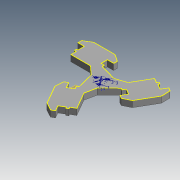
# Autodesk Inventor part: Part2
Saved by Autodesk Inventor 2014 SP1 (Build 180222100, 222)
## iProperties
Created: 2014-04-03
Part Number: Part2
Material: Generic
Document SubType Name: Modeling
Designer: tom
Density: 1 g/cm^3
Appearance: Default
Author: tom
Autodesk Inventor part; units mm, degrees
ref_plane "YZ Plane" through (0, 0, 0) normal (1, 0, 0) x (0, 1, 0)
ref_plane "XZ Plane" through (0, 0, 0) normal (0, 1, 0) x (-1, 0, 0)
ref_plane "XY Plane" through (0, 0, 0) normal (0, 0, 1) x (1, 0, 0)
ref_plane "Work Plane3" through (-98.2192, 25.6748, -72.651) normal (0, 1, 0) x (1, 0, 0)
sketch "Sketch1" plane through (-98.2192, 25.6748, -72.651) normal (0, 1, 0) x (1, 0, 0)
  line L0 (108.2722, -112.7231) -> (109.1382, -112.2231) construction
  line L1 (108.6382, -111.3571) -> (109.1382, -112.2231) construction
  line L2 (101.5917, -99.1522) -> (114.8917, -122.1885)
  line L3 (114.8917, -122.1885) -> (108.6563, -125.7885)
  line L4 (108.6563, -125.7885) -> (109.9613, -128.0488)
  line L5 (109.9613, -128.0488) -> (107.3632, -129.5488)
  line L6 (107.3632, -129.5488) -> (106.3632, -127.8168)
  line L7 (106.3632, -127.8168) -> (98.8635, -132.1468)
  line L8 (98.8635, -132.1468) -> (103.1935, -139.6466)
  line L9 (79.4712, -121.2385) -> (82.4842, -126.4571) construction
  line L10 (103.1935, -139.6466) -> (98.8633, -142.1466)
  line L11 (83.0235, -104.7111) -> (90.5232, -100.3811)
  line L12 (90.5232, -100.3811) -> (88.3182, -96.5619)
  line L13 (88.3182, -96.5619) -> (90.8427, -95.1044)
  line L14 (83.0235, -104.7111) -> (78.6935, -97.2113)
  line L15 (73.6327, -111.1259) -> (88.2377, -136.4225)
  line L16 (78.6935, -97.2113) -> (74.3633, -99.7113)
  line L17 (90.8427, -95.1044) -> (85.0892, -72.651)
  line L18 (104.7842, -84.0219) -> (98.2192, -72.651)
  line L19 (98.2192, -72.651) -> (85.0892, -72.651)
  line L20 (88.2377, -136.4225) -> (98.8633, -142.1466)
  line L21 (74.3633, -99.7113) -> (73.6327, -111.1259)
  line L22 (98.2192, -72.651) -> (104.7842, -84.0219)
  line L23 (104.7842, -84.0219) -> (101.5917, -99.1522)
  dimension "d1" = 26.6
  dimension "d4" = 7.2
  dimension "d5" = 2.61
  dimension "d6" = 3
  dimension "d7" = 2
  dimension "d8" = 8.66
  dimension "d9" = 8.66
  dimension "d10" = 5
  dimension "d11" = 8.66
  dimension "d12" = 31.68
  dimension "d13" = 4.41
  dimension "d14" = 2.915
  dimension "d17" = 8.66
  dimension "d18" = 29.21
  dimension "d20" = 10.27
  dimension "d21" = 5
  dimension "d22" = 23.1789
  dimension "d23" = 13.13
  dimension "d31" = 13.13
  constraints: 48 end point, 7 perpendicular, 1 collinear, 1 parallel
  measures "d1" distance of L2.start L2.end
  measures "d4" distance of L2.end L3.end
  measures "d5" distance of L3.end L4.end
  measures "d6" distance of L4.end L5.end
  measures "d7" distance of L5.end L6.end
  measures "d8" distance of L6.end L7.end
  measures "d9" distance of L7.end L8.end
  measures "d10" distance of L8.end L10.end
  measures "d11" distance of L11.start L11.end
  measures "d12" distance between parallel lines of L7 L11
  measures "d13" distance of L11.end L12.end
  measures "d14" distance of L12.end L13.end
  measures "d17" distance of L11.start L14.end
  measures "d18" distance of L15.start L15.end
  measures "d20" distance from line of L10 L15.end
  measures "d21" distance of L14.end L16.end
  measures "d22" distance of L13.end L17.end
  measures "d23" distance of L18.end L17.end
  measures "d31" distance of L18.start L18.end
extrude "Extrusion1" add sketch "Sketch1" along normal blind 8.66
pattern_circular "Circular Pattern2" count 3 over 360 about axis through (0, 25.6748, 0) along (0, 1, 0) of "Extrusion1"
sketch "Sketch2" plane through (-98.2192, 34.3348, -72.651) normal (0, 1, 0) x (1, 0, 0)
  line L0 (46.9822, -62.321) -> (73.5822, -62.321) projected
  line L1 (114.8917, -122.1885) -> (101.5917, -99.1522) projected
  circle A0 centre (98.2192, -72.651) radius 1.5
  line L2 (98.2192, -72.651) -> (104.7842, -84.0219) construction
  line L3 (98.2192, -72.651) -> (85.0892, -72.651) construction
  line L4 (98.2192, -72.651) -> (104.7842, -61.28) construction
  circle A1 centre (98.2192, -72.651) radius 7 construction
  circle A2 centre (101.7192, -78.7131) radius 1.5
  circle A3 centre (101.7192, -66.5888) radius 1.5
  circle A4 centre (91.2192, -72.651) radius 1.5
  dimension "d35" = 3
  dimension "d36" = 14
  dimension "d37" = 3
  dimension "d38" = 3
  dimension "d39" = 3
  constraints: 6 end point, 5 centre point, 3 point on circle, 3 point on line, 2 coincident, 2 parallel
  measures "d35" diameter of A0
  measures "d36" diameter of A1
  measures "d37" diameter of A2
  measures "d38" diameter of A3
  measures "d39" diameter of A4
extrude "Extrusion2" cut sketch "Sketch2" against normal blind 10
body "Solid1"
